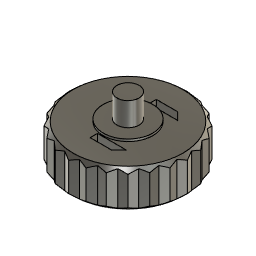
secondary_015mm_wheel (Autodesk Fusion 360 design; units mm, degrees)
Autodesk Fusion 360 part; units mm, degrees
other "Base Mesh Feature1"
sketch "Sketch1" plane through (0, 0, 0) normal (0, 0, 1) x (1, 0, 0)
  circle A0 centre (0, 0) radius 1
  dimension "d1" = 2
  constraint coincident A0.centre origin
  measures "d1" diameter of A0
other "Modify1"
other "Modify2"
sketch "Sketch2" plane through (0, 0, 0) normal (0, 0, 1) x (1, 0, 0)
  line L0 (0, -10.7634) -> (-1.3413, -10.1465)
  line L1 (0, -10.7634) -> (1.3687, -10.1568)
  line L2 (1.3687, -10.1568) -> (1.3687, -10.1544)
  line L3 (2.7858, -10.3966) -> (1.3305, -10.1479)
  line L4 (2.7858, -10.3966) -> (3.9508, -9.4565)
  line L5 (3.9508, -9.4565) -> (3.9502, -9.4542)
  line L6 (5.3817, -9.3214) -> (3.9116, -9.4578)
  line L7 (5.3817, -9.3214) -> (6.2637, -8.1117)
  line L8 (6.2637, -8.1117) -> (6.2625, -8.1096)
  line L9 (7.6109, -7.6109) -> (6.2262, -8.1231)
  line L10 (7.6109, -7.6109) -> (8.1497, -6.2141)
  line L11 (8.1497, -6.2141) -> (8.1481, -6.2125)
  line L12 (9.3214, -5.3817) -> (8.1164, -6.2348)
  line L13 (9.3214, -5.3817) -> (9.4804, -3.8931)
  line L14 (9.4804, -3.8931) -> (9.4783, -3.8919)
  line L15 (10.3966, -2.7858) -> (9.4536, -3.9217)
  line L16 (10.3966, -2.7858) -> (10.165, -1.3067)
  line L17 (10.165, -1.3067) -> (10.1627, -1.3061)
  line L18 (10.7634, 0) -> (10.1465, -1.3413)
  line L19 (10.7634, 0) -> (10.1568, 1.3687)
  line L20 (10.1568, 1.3687) -> (10.1544, 1.3687)
  line L21 (10.3966, 2.7858) -> (10.1479, 1.3305)
  line L22 (10.3966, 2.7858) -> (9.4565, 3.9508)
  line L23 (9.4565, 3.9508) -> (9.4542, 3.9502)
  line L24 (9.3214, 5.3817) -> (9.4578, 3.9116)
  line L25 (9.3214, 5.3817) -> (8.1117, 6.2637)
  line L26 (8.1117, 6.2637) -> (8.1096, 6.2625)
  line L27 (7.6109, 7.6109) -> (8.1231, 6.2262)
  line L28 (7.6109, 7.6109) -> (6.2141, 8.1497)
  line L29 (6.2141, 8.1497) -> (6.2125, 8.1481)
  line L30 (5.3817, 9.3214) -> (6.2348, 8.1164)
  line L31 (5.3817, 9.3214) -> (3.8931, 9.4804)
  line L32 (3.8931, 9.4804) -> (3.8919, 9.4783)
  line L33 (2.7858, 10.3966) -> (3.9217, 9.4536)
  line L34 (2.7858, 10.3966) -> (1.3067, 10.165)
  line L35 (1.3067, 10.165) -> (1.3061, 10.1627)
  line L36 (0, 10.7634) -> (1.3413, 10.1465)
  line L37 (0, 10.7634) -> (-1.3687, 10.1568)
  line L38 (-1.3687, 10.1568) -> (-1.3687, 10.1544)
  line L39 (-2.7858, 10.3966) -> (-1.3305, 10.1479)
  line L40 (-2.7858, 10.3966) -> (-3.9508, 9.4565)
  line L41 (-3.9508, 9.4565) -> (-3.9502, 9.4542)
  line L42 (-5.3817, 9.3214) -> (-3.9116, 9.4578)
  line L43 (-5.3817, 9.3214) -> (-6.2637, 8.1117)
  line L44 (-6.2637, 8.1117) -> (-6.2625, 8.1096)
  line L45 (-7.6109, 7.6109) -> (-6.2262, 8.1231)
  line L46 (-7.6109, 7.6109) -> (-8.1497, 6.2141)
  line L47 (-8.1497, 6.2141) -> (-8.1481, 6.2125)
  line L48 (-9.3214, 5.3817) -> (-8.1164, 6.2348)
  line L49 (-9.3214, 5.3817) -> (-9.4804, 3.8931)
  line L50 (-9.4804, 3.8931) -> (-9.4783, 3.8919)
  line L51 (-10.3966, 2.7858) -> (-9.4536, 3.9217)
  line L52 (-10.3966, 2.7858) -> (-10.165, 1.3067)
  line L53 (-10.165, 1.3067) -> (-10.1627, 1.3061)
  line L54 (-10.7634, 0) -> (-10.1465, 1.3413)
  line L55 (-10.7634, 0) -> (-10.1568, -1.3687)
  line L56 (-10.1568, -1.3687) -> (-10.1544, -1.3687)
  line L57 (-10.3966, -2.7858) -> (-10.1479, -1.3305)
  line L58 (-10.3966, -2.7858) -> (-9.4565, -3.9508)
  line L59 (-9.4565, -3.9508) -> (-9.4542, -3.9502)
  line L60 (-9.3214, -5.3817) -> (-9.4578, -3.9116)
  line L61 (-9.3214, -5.3817) -> (-8.1117, -6.2637)
  line L62 (-8.1117, -6.2637) -> (-8.1096, -6.2625)
  line L63 (-7.6109, -7.6109) -> (-8.1231, -6.2262)
  line L64 (-7.6109, -7.6109) -> (-6.2141, -8.1497)
  line L65 (-6.2141, -8.1497) -> (-6.2125, -8.1481)
  line L66 (-5.3817, -9.3214) -> (-6.2348, -8.1164)
  line L67 (-5.3817, -9.3214) -> (-3.8931, -9.4804)
  line L68 (-3.8931, -9.4804) -> (-3.8919, -9.4783)
  line L69 (-2.7858, -10.3966) -> (-3.9217, -9.4536)
  line L70 (-2.7858, -10.3966) -> (-1.3067, -10.165)
  line L71 (-1.3067, -10.165) -> (-1.3061, -10.1627)
  line L72 (-0.8666, -5.9914) -> (-0.8666, 6)
  line L73 (-0.8666, 6) -> (3, 6)
  line L74 (3, 6) -> (6, 3)
  line L75 (6, 3) -> (6, -3)
  line L76 (6, -3) -> (3, -6)
  line L77 (3, -6) -> (-0.8666, -5.9914)
  constraint vertical L2
  constraint coincident L69 L68.end
  constraint coincident L0 L71.end
  constraint coincident L3 L2.end
  constraint coincident L6 L5.end
  constraint coincident L9 L8.end
  constraint coincident L12 L11.end
  constraint coincident L15 L14.end
  constraint coincident L18 L17.end
  constraint coincident L21 L20.end
  constraint coincident L24 L23.end
  constraint coincident L27 L26.end
  constraint coincident L30 L29.end
  constraint coincident L33 L32.end
  constraint coincident L36 L35.end
  constraint coincident L39 L38.end
  constraint coincident L42 L41.end
  constraint coincident L45 L44.end
  constraint coincident L48 L47.end
  constraint coincident L51 L50.end
  constraint coincident L54 L53.end
  constraint coincident L57 L56.end
  constraint coincident L60 L59.end
  constraint coincident L63 L62.end
  constraint coincident L66 L65.end
  constraint vertical L72
  constraint perpendicular L72 L73
  constraint parallel L72 L75
  constraint perpendicular L74 L76
extrude "Extrude1" add sketch "Sketch2" along normal blind 6.75 contours L0 L1 L2 L3 L4 L5 L6 L7 L8 L9 L10 L11 L12 L13 L14 L15 L16 L17 L18 L19 L20 L21 L22 L23 L24 L25 L26 L27 L28 L29 L30 L31 L32 L33 L34 L35 L36 L37 L38 L39 L40 L41 L42 L43 L44 L45 L46 L47 L48 L49 L50 L51 L52 L53 L54 L55 L56 L57 L58 L59 L60 L61 L62 L63 L64 L65 L66 L67 L68 L69 L70 L71 makes body 1
sketch "Sketch3" plane through (0, 0, 6.75) normal (0, 0, 1) x (-1, 0, 0)
  line L0 (-6, 3) -> (-3, 6)
  line L1 (-3, 6) -> (0.8666, 5.9914)
  line L2 (0.8666, 5.9914) -> (0.8666, -6)
  line L3 (0.8666, -6) -> (-3, -6)
  line L4 (-3, -6) -> (-6, -3)
  line L5 (-6, -3) -> (-6, 3)
  line L6 (2.7858, 10.3966) -> (1.3067, 10.165)
  line L7 (1.3067, 10.165) -> (1.3061, 10.1627)
  line L8 (1.3061, 10.1627) -> (0, 10.7634)
  line L9 (0, 10.7634) -> (-1.3687, 10.1568)
  line L10 (-1.3687, 10.1568) -> (-1.3687, 10.1544)
  line L11 (-1.3687, 10.1544) -> (-2.7858, 10.3966)
  line L12 (-2.7858, 10.3966) -> (-3.9508, 9.4565)
  line L13 (-3.9508, 9.4565) -> (-3.9502, 9.4542)
  line L14 (-3.9502, 9.4542) -> (-5.3817, 9.3214)
  line L15 (-5.3817, 9.3214) -> (-6.2637, 8.1117)
  line L16 (-6.2637, 8.1117) -> (-6.2625, 8.1096)
  line L17 (-6.2625, 8.1096) -> (-7.6109, 7.6109)
  line L18 (-7.6109, 7.6109) -> (-8.1497, 6.2141)
  line L19 (-8.1497, 6.2141) -> (-8.1481, 6.2125)
  line L20 (-8.1481, 6.2125) -> (-9.3214, 5.3817)
  line L21 (-9.3214, 5.3817) -> (-9.4804, 3.8931)
  line L22 (-9.4804, 3.8931) -> (-9.4783, 3.8919)
  line L23 (-9.4783, 3.8919) -> (-10.3966, 2.7858)
  line L24 (-10.3966, 2.7858) -> (-10.165, 1.3067)
  line L25 (-10.165, 1.3067) -> (-10.1627, 1.3061)
  line L26 (-10.1627, 1.3061) -> (-10.7634, 0)
  line L27 (-10.7634, 0) -> (-10.1568, -1.3687)
  line L28 (-10.1568, -1.3687) -> (-10.1544, -1.3687)
  line L29 (-10.1544, -1.3687) -> (-10.3966, -2.7858)
  line L30 (-10.3966, -2.7858) -> (-9.4565, -3.9508)
  line L31 (-9.4565, -3.9508) -> (-9.4542, -3.9502)
  line L32 (-9.4542, -3.9502) -> (-9.3214, -5.3817)
  line L33 (-9.3214, -5.3817) -> (-8.1117, -6.2637)
  line L34 (-8.1117, -6.2637) -> (-8.1096, -6.2625)
  line L35 (-8.1096, -6.2625) -> (-7.6109, -7.6109)
  line L36 (-7.6109, -7.6109) -> (-6.2141, -8.1497)
  line L37 (-6.2141, -8.1497) -> (-6.2125, -8.1481)
  line L38 (-6.2125, -8.1481) -> (-5.3817, -9.3214)
  line L39 (-5.3817, -9.3214) -> (-3.8931, -9.4804)
  line L40 (-3.8931, -9.4804) -> (-3.8919, -9.4783)
  line L41 (-3.8919, -9.4783) -> (-2.7858, -10.3966)
  line L42 (-2.7858, -10.3966) -> (-1.3067, -10.165)
  line L43 (-1.3067, -10.165) -> (-1.3061, -10.1627)
  line L44 (-1.3061, -10.1627) -> (0, -10.7634)
  line L45 (0, -10.7634) -> (1.3687, -10.1568)
  line L46 (1.3687, -10.1568) -> (1.3687, -10.1544)
  line L47 (1.3687, -10.1544) -> (2.7858, -10.3966)
  line L48 (2.7858, -10.3966) -> (3.9508, -9.4565)
  line L49 (3.9508, -9.4565) -> (3.9502, -9.4542)
  line L50 (3.9502, -9.4542) -> (5.3817, -9.3214)
  line L51 (5.3817, -9.3214) -> (6.2637, -8.1117)
  line L52 (6.2637, -8.1117) -> (6.2625, -8.1096)
  line L53 (6.2625, -8.1096) -> (7.6109, -7.6109)
  line L54 (7.6109, -7.6109) -> (8.1497, -6.2141)
  line L55 (8.1497, -6.2141) -> (8.1481, -6.2125)
  line L56 (8.1481, -6.2125) -> (9.3214, -5.3817)
  line L57 (9.3214, -5.3817) -> (9.4804, -3.8931)
  line L58 (9.4804, -3.8931) -> (9.4783, -3.8919)
  line L59 (9.4783, -3.8919) -> (10.3966, -2.7858)
  line L60 (10.3966, -2.7858) -> (10.165, -1.3067)
  line L61 (10.165, -1.3067) -> (10.1627, -1.3061)
  line L62 (10.1627, -1.3061) -> (10.7634, 0)
  line L63 (10.7634, 0) -> (10.1568, 1.3687)
  line L64 (10.1568, 1.3687) -> (10.1544, 1.3687)
  line L65 (10.1544, 1.3687) -> (10.3966, 2.7858)
  line L66 (10.3966, 2.7858) -> (9.4565, 3.9508)
  line L67 (9.4565, 3.9508) -> (9.4542, 3.9502)
  line L68 (9.4542, 3.9502) -> (9.3214, 5.3817)
  line L69 (9.3214, 5.3817) -> (8.1117, 6.2637)
  line L70 (8.1117, 6.2637) -> (8.1096, 6.2625)
  line L71 (8.1096, 6.2625) -> (7.6109, 7.6109)
  line L72 (7.6109, 7.6109) -> (6.2141, 8.1497)
  line L73 (6.2141, 8.1497) -> (6.2125, 8.1481)
  line L74 (6.2125, 8.1481) -> (5.3817, 9.3214)
  line L75 (5.3817, 9.3214) -> (3.8931, 9.4804)
  line L76 (3.8931, 9.4804) -> (3.8919, 9.4783)
  line L77 (3.8919, 9.4783) -> (2.7858, 10.3966)
  circle A0 centre (0, 0) radius 4.5023
  constraint coincident A0.centre origin
ref_plane "WorkPlane1" through (0, -4.5, 0) normal (0, 1, 0) x (0, 0, 1)
sketch "Sketch4" plane through (-0.8666, 0, 0) normal (1, 0, 0) x (0, 1, 0)
  line L0 (-5.9914, 0) -> (6, 0)
  line L1 (6, 0) -> (6, 6.75)
  line L2 (6, 6.75) -> (-5.9914, 6.75)
  line L3 (-5.9914, 6.75) -> (-5.9914, 0)
  line L4 (-4.663, 6.75) -> (4.637, 6.75)
  line L5 (4.637, 6.75) -> (4.637, 4.75)
  line L6 (4.637, 4.75) -> (-4.663, 4.75)
  line L7 (-4.663, 4.75) -> (-4.663, 6.75)
  dimension "d7" = 9.3
  dimension "d8" = 2
  constraint horizontal L4
  constraint vertical L5
  constraint horizontal L6
  constraint vertical L7
  constraint coincident L2 L4.start
  measures "d7" distance of L4.start L4.end
  measures "d8" distance of L4.start L6.end
extrude "Extrude2" add sketch "Sketch4" along normal blind 7.5 contours L2 L4 L5 L6 L7 bodies 1
extrude "Extrude3" add sketch "Sketch3" along normal blind 0.4 contours L2 A0 | L2 A0 bodies 1
sketch "Sketch5" plane through (0, 0, 7.15) normal (0, 0, 1) x (-1, 0, 0)
  circle A0 centre (0, 0) radius 4.5023
  circle A1 centre (0, 0) radius 2
  dimension "d13" = 4
  constraint concentric A0 A1
  measures "d13" diameter of A1
extrude "Extrude4" add sketch "Sketch5" along normal blind 4.25 contours A1 bodies 1
sketch "Sketch6" plane through (0, 0, 0) normal (0, 1, 0) x (1, 0, 0)
  line L0 (9.7, -7) -> (11, -5.8)
  line L1 (11, -5.8) -> (11, -7)
  line L2 (11, -7) -> (9.7, -7)
  line L3 (11, 0.2) -> (9.7, 0.2)
  line L4 (11, -1) -> (11, 0.2)
  line L5 (9.7, 0.2) -> (11, -1)
  line L6 (11, 0.2) -> (9.7, 0.2)
  constraint vertical L1
  constraint perpendicular L1 L2
  constraint symmetric L4.end L3 L6.start
  constraint symmetric L5.start L3 L6.end
revolve "Revolve1" cut sketch "Sketch6" angle 360 about axis through (0, 0, 1.75) along (0, 0, 1) contours L0 L1 L2 bodies 1
revolve "Revolve2" cut sketch "Sketch6" angle 360 about axis through (0, 0, 1.75) along (0, 0, 1) contours L3 L4 L5 L6 bodies 1
copy_body "Body->Comp1" bodies 1 removing the originals makes body 2 in component "secondary_015mm_wheel"
component "secondary_015mm_wheel" placed x (1, 0, 0) y (0, 1, 0) z (0, 0, 1) at (0, 0, 0)
named bodies: "secondary_015mm_wheel (1)"
